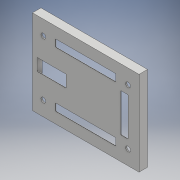
# Autodesk Inventor part: Platform-top
Saved by Autodesk Inventor 2017 (Build 210142000, 142)
## iProperties
Created: 2018-03-19
Part Number: Platform-top
Material: Generic
Document SubType Name: Modeling
Designer: Arjuna
Density: 1 g/cm^3
Appearance: Default
Author: Arjuna
Autodesk Inventor part; units mm, degrees
ref_plane "YZ Plane" through (0, 0, 0) normal (1, 0, 0) x (0, 1, 0)
ref_plane "XZ Plane" through (0, 0, 0) normal (0, 1, 0) x (-1, 0, 0)
ref_plane "XY Plane" through (0, 0, 0) normal (0, 0, 1) x (1, 0, 0)
sketch "Sketch1" plane through (0, 0, 0) normal (0, 1, 0) x (-1, 0, 0)
  line L0 (109.5, 87) -> (-109.5, 87)
  line L1 (-109.5, 87) -> (-109.5, -87)
  line L2 (-109.5, -87) -> (109.5, -87)
  line L3 (109.5, -87) -> (109.5, 87)
  point P0 (0, 0)
  dimension "d0" = 219
  dimension "d1" = 174
  dimension "d2" = 87
  dimension "d3" = 109.5
  constraints: 8 end point, 2 parallel, 1 horizontal, 1 perpendicular
  measures "d0" distance of L1.end L2.end
  measures "d1" distance of L2.end L0.start
  measures "d2" distance from line of point (0, 0) L0
  measures "d3" distance from line of point (0, 0) L1
extrude "Extrusion1" add sketch "Sketch1" along normal blind 17.5
sketch "Sketch2" plane through (0, 17.5, 0) normal (0, 1, 0) x (1, 0, 0)
  line L0 (-109.5, -87) -> (109.5, -87) projected
  line L1 (109.5, -87) -> (109.5, 87) projected
  line L2 (109.5, 87) -> (-109.5, 87) projected
  line L3 (-109.5, 87) -> (-109.5, -87) projected
  line L4 (-107, -84.5) -> (107, -84.5)
  line L5 (107, -84.5) -> (107, 84.5)
  line L6 (107, 84.5) -> (-107, 84.5)
  line L7 (-107, 84.5) -> (-107, -84.5)
  point P0 (0, 0)
  dimension "d6" = 2.5
  dimension "d7" = 2.5
  dimension "d8" = 2.5
  dimension "d9" = 2.5
  constraints: 8 end point, 2 parallel, 1 horizontal, 1 perpendicular
  measures "d6" distance between parallel lines of L3 L7
  measures "d7" distance between parallel lines of L2 L6
  measures "d8" distance between parallel lines of L0 L4
  measures "d9" distance between parallel lines of L1 L5
extrude "Extrusion2" cut sketch "Sketch2" against normal blind 15 contours L7 L6 L5 L4
sketch "Sketch3" plane through (0, 2.5, 0) normal (0, 1, 0) x (1, 0, 0)
  line L0 (-100, -12.5) -> (-40, -12.5)
  line L1 (-40, -12.5) -> (-40, 12.5)
  line L2 (-40, 12.5) -> (-100, 12.5)
  line L3 (-100, 12.5) -> (-100, -12.5)
  line L4 (-50, -19.5594) -> (-50, 30.4406)
  point P0 (0, 0)
  dimension "d12" = 60
  dimension "d13" = 25
  dimension "d14" = 12.5
  dimension "d15" = 40
  dimension "d16" = 50
  dimension "d17" = 50
  dimension "d18" = 50
  constraints: 10 end point, 2 parallel, 1 horizontal, 1 perpendicular, 1 vertical
  measures "d12" distance of L2.end L1.end
  measures "d13" distance of L2.end L0.start
  measures "d14" distance from line of point (0, 0) L0
  measures "d15" distance from line of point (0, 0) L1
  measures "d16" distance of L4.start L4.end
  measures "d17" distance from line of point (0, 0) L4
  measures "d18" distance between parallel lines of L4 L3
extrude "Extrusion3" cut sketch "Sketch3" against normal through all
sketch "Sketch4" plane through (0, 2.5, 0) normal (0, 1, 0) x (1, 0, 0)
  line L0 (-87, -64.5) -> (87, -64.5)
  line L1 (87, -64.5) -> (87, 64.5)
  line L2 (87, 64.5) -> (-87, 64.5)
  line L3 (-87, 64.5) -> (-87, -64.5)
  line L4 (-40, 12.5) -> (-40, -12.5) projected
  line L5 (-40, -12.5) -> (-100, -12.5) projected
  line L6 (-100, -12.5) -> (-100, 12.5) projected
  line L7 (-100, 12.5) -> (-40, 12.5) projected
  line L8 (107, -84.5) -> (-107, -84.5) projected
  line L9 (107, 84.5) -> (107, -84.5) projected
  line L10 (-107, 84.5) -> (107, 84.5) projected
  line L11 (-107, -84.5) -> (-107, 84.5) projected
  line L12 (-72, -49.5) -> (72, -49.5)
  line L13 (72, -49.5) -> (72, 49.5)
  line L14 (72, 49.5) -> (-72, 49.5)
  line L15 (-72, 49.5) -> (-72, -49.5)
  line L16 (-87, -39.5) -> (-72, -39.5)
  line L17 (-62, -49.5) -> (-62, -64.5)
  line L18 (-72, 39.5) -> (-87, 39.5)
  line L19 (-62, 49.5) -> (-62, 64.5)
  line L20 (62, 49.5) -> (62, 64.5)
  line L21 (72, 39.5) -> (87, 39.5)
  line L22 (72, -39.5) -> (87, -39.5)
  line L23 (62, -49.5) -> (62, -64.5)
  point P0 (0, 0)
  dimension "d21" = 20
  dimension "d22" = 20
  dimension "d23" = 20
  dimension "d24" = 20
  dimension "d25" = 15
  dimension "d26" = 15
  dimension "d27" = 15
  dimension "d28" = 15
  dimension "d29" = 25
  dimension "d30" = 25
  dimension "d31" = 25
  dimension "d32" = 25
  dimension "d33" = 25
  dimension "d34" = 25
  dimension "d35" = 25
  dimension "d36" = 25
  dimension "d169" = 129
  dimension "d170" = 174
  dimension "d171" = 87
  dimension "d172" = 64.5
  constraints: 32 end point, 16 point on line, 10 perpendicular, 4 parallel, 2 horizontal
  measures "d21" distance between parallel lines of L3 L11
  measures "d22" distance between parallel lines of L8 L0
  measures "d23" distance between parallel lines of L10 L2
  measures "d24" distance between parallel lines of L9 L1
  measures "d25" distance between parallel lines of L15 L3
  measures "d26" distance between parallel lines of L2 L14
  measures "d27" distance between parallel lines of L0 L12
  measures "d28" distance between parallel lines of L1 L13
  measures "d29" distance between parallel lines of L0 L16
  measures "d30" distance between parallel lines of L3 L17
  measures "d31" distance between parallel lines of L2 L18
  measures "d32" distance between parallel lines of L19 L3
  measures "d33" distance between parallel lines of L1 L20
  measures "d34" distance between parallel lines of L2 L21
  measures "d35" distance between parallel lines of L1 L23
  measures "d36" distance between parallel lines of L22 L0
  measures "d169" distance of L2.end L0.start
  measures "d170" distance of L0.start L0.end
  measures "d171" distance from line of point (0, 0) L3
  measures "d172" distance from line of point (0, 0) L0
extrude "Extrusion4" cut sketch "Sketch4" against normal through all contours L17 L12 L23 L0 | L22 L13 L21 L1 | L2 L20 L14 L19
sketch "Sketch5" plane through (0, 2.5, 0) normal (0, 1, 0) x (1, 0, 0)
  line L0 (62, -64.5) -> (-62, -64.5) projected
  line L1 (-62, -64.5) -> (-62, -49.5) projected
  line L2 (-62, -49.5) -> (62, -49.5) projected
  line L3 (62, -49.5) -> (62, -64.5) projected
  line L4 (87, -39.5) -> (72, -39.5) projected
  line L5 (72, -39.5) -> (72, 39.5) projected
  line L6 (72, 39.5) -> (87, 39.5) projected
  line L7 (87, 39.5) -> (87, -39.5) projected
  line L8 (62, 64.5) -> (62, 49.5) projected
  line L9 (62, 49.5) -> (-62, 49.5) projected
  line L10 (-62, 49.5) -> (-62, 64.5) projected
  line L11 (-62, 64.5) -> (62, 64.5) projected
  line L12 (-40, 12.5) -> (-40, -12.5) projected
  line L13 (-40, -12.5) -> (-100, -12.5) projected
  line L14 (-100, -12.5) -> (-100, 12.5) projected
  line L15 (-100, 12.5) -> (-40, 12.5) projected
  line L16 (107, -84.5) -> (-107, -84.5) projected
  line L17 (107, 84.5) -> (107, -84.5) projected
  line L18 (-107, 84.5) -> (107, 84.5) projected
  line L19 (-107, -84.5) -> (-107, 84.5) projected
  line L20 (-62, -62) -> (-72, -62)
  line L21 (-72, -62) -> (-72, -52)
  line L22 (-72, -52) -> (-62, -52)
  line L23 (-62, -52) -> (-62, -62)
  line L24 (62, -62) -> (72, -62)
  line L25 (72, -62) -> (72, -52)
  line L26 (72, -52) -> (62, -52)
  line L27 (62, -52) -> (62, -62)
  line L28 (84.5, -39.5) -> (74.5, -39.5)
  line L29 (74.5, -39.5) -> (74.5, -49.5)
  line L30 (74.5, -49.5) -> (84.5, -49.5)
  line L31 (84.5, -49.5) -> (84.5, -39.5)
  line L32 (74.5, 39.5) -> (84.5, 39.5)
  line L33 (84.5, 39.5) -> (84.5, 49.5)
  line L34 (84.5, 49.5) -> (74.5, 49.5)
  line L35 (74.5, 49.5) -> (74.5, 39.5)
  line L36 (-62, 52) -> (-72, 52)
  line L37 (-72, 52) -> (-72, 62)
  line L38 (-72, 62) -> (-62, 62)
  line L39 (-62, 62) -> (-62, 52)
  line L40 (62, 52) -> (72, 52)
  line L41 (72, 52) -> (72, 62)
  line L42 (72, 62) -> (62, 62)
  line L43 (62, 62) -> (62, 52)
  line L44 (-40, -10) -> (-30, -10)
  line L45 (-30, -10) -> (-30, 5)
  line L46 (-30, 5) -> (-40, 5)
  line L47 (-40, 5) -> (-40, -10)
  line L48 (-95, 12.5) -> (-45, 12.5)
  line L49 (-45, 12.5) -> (-45, 22.5)
  line L50 (-45, 22.5) -> (-95, 22.5)
  line L51 (-95, 22.5) -> (-95, 12.5)
  line L52 (-95, -12.5) -> (-45, -12.5)
  line L53 (-45, -12.5) -> (-45, -22.5)
  line L54 (-45, -22.5) -> (-95, -22.5)
  line L55 (-95, -22.5) -> (-95, -12.5)
  line L56 (-50, -49.5) -> (50, -49.5)
  line L57 (50, -49.5) -> (50, -39.5)
  line L58 (50, -39.5) -> (-50, -39.5)
  line L59 (-50, -39.5) -> (-50, -49.5)
  line L60 (-50, -64.5) -> (50, -64.5)
  line L61 (50, -64.5) -> (50, -74.5)
  line L62 (50, -74.5) -> (-50, -74.5)
  line L63 (-50, -74.5) -> (-50, -64.5)
  line L64 (-50, 49.5) -> (50, 49.5)
  line L65 (50, 49.5) -> (50, 39.5)
  line L66 (50, 39.5) -> (-50, 39.5)
  line L67 (-50, 39.5) -> (-50, 49.5)
  line L68 (-50, 64.5) -> (50, 64.5)
  line L69 (50, 64.5) -> (50, 74.5)
  line L70 (50, 74.5) -> (-50, 74.5)
  line L71 (-50, 74.5) -> (-50, 64.5)
  line L72 (72, -32.5) -> (62, -32.5)
  line L73 (62, -32.5) -> (62, 32.5)
  line L74 (62, 32.5) -> (72, 32.5)
  line L75 (72, 32.5) -> (72, -32.5)
  line L76 (87, -32.5) -> (97, -32.5)
  line L77 (97, -32.5) -> (97, 32.5)
  line L78 (97, 32.5) -> (87, 32.5)
  line L79 (87, 32.5) -> (87, -32.5)
  point P0 (0, 0)
  dimension "d39" = 10
  dimension "d40" = 10
  dimension "d41" = 2.5
  dimension "d42" = 2.5
  dimension "d43" = 10
  dimension "d44" = 10
  dimension "d45" = 2.5
  dimension "d46" = 2.5
  dimension "d47" = 10
  dimension "d48" = 10
  dimension "d49" = 2.5
  dimension "d50" = 2.5
  dimension "d51" = 10
  dimension "d52" = 10
  dimension "d53" = 2.5
  dimension "d54" = 2.5
  dimension "d55" = 10
  dimension "d56" = 10
  dimension "d57" = 2.5
  dimension "d58" = 10
  dimension "d59" = 10
  dimension "d60" = 2.5
  dimension "d61" = 2.5
  dimension "d62" = 10
  dimension "d63" = 15
  dimension "d64" = 2.5
  dimension "d65" = 7.5
  dimension "d66" = 50
  dimension "d67" = 10
  dimension "d68" = 5
  dimension "d69" = 5
  dimension "d70" = 50
  dimension "d71" = 10
  dimension "d72" = 5
  dimension "d73" = 5
  dimension "d74" = 100
  dimension "d75" = 10
  dimension "d76" = 12
  dimension "d77" = 12
  dimension "d78" = 100
  dimension "d79" = 10
  dimension "d80" = 12
  dimension "d81" = 12
  dimension "d82" = 100
  dimension "d83" = 10
  dimension "d84" = 12
  dimension "d85" = 12
  dimension "d86" = 100
  dimension "d87" = 10
  dimension "d88" = 12
  dimension "d89" = 12
  dimension "d90" = 65
  dimension "d91" = 10
  dimension "d92" = 7
  dimension "d93" = 7
  dimension "d94" = 10
  dimension "d95" = 65
  dimension "d96" = 7
  dimension "d97" = 7
  constraints: 120 end point, 30 parallel, 15 horizontal, 15 perpendicular, 15 point on line
  measures "d39" distance of L21.end L22.end
  measures "d40" distance of L20.end L21.end
  measures "d41" distance between parallel lines of L2 L22
  measures "d42" distance between parallel lines of L20 L0
  measures "d43" distance of L30.end L29.end
  measures "d44" distance of L28.end L29.end
  measures "d45" distance between parallel lines of L29 L5
  measures "d46" distance between parallel lines of L7 L31
  measures "d47" distance of L25.end L26.end
  measures "d48" distance of L24.end L25.end
  measures "d49" distance between parallel lines of L24 L0
  measures "d50" distance between parallel lines of L2 L26
  measures "d51" distance of L34.end L32.start
  measures "d52" distance of L33.end L34.end
  measures "d53" distance between parallel lines of L35 L5
  measures "d54" distance between parallel lines of L33 L7
  measures "d55" distance of L36.end L37.end
  measures "d56" distance of L37.end L38.end
  measures "d57" distance between parallel lines of L36 L9
  measures "d58" distance of L40.end L41.end
  measures "d59" distance of L41.end L42.end
  measures "d60" distance between parallel lines of L40 L9
  measures "d61" distance between parallel lines of L11 L42
  measures "d62" distance of L46.end L45.end
  measures "d63" distance of L44.end L45.end
  measures "d64" distance between parallel lines of L44 L13
  measures "d65" distance between parallel lines of L15 L46
  measures "d66" distance of L50.end L49.end
  measures "d67" distance of L50.end L48.start
  measures "d68" distance between parallel lines of L49 L12
  measures "d69" distance between parallel lines of L51 L14
  measures "d70" distance of L53.end L54.end
  measures "d71" distance of L54.end L52.start
  measures "d72" distance between parallel lines of L12 L53
  measures "d73" distance between parallel lines of L14 L55
  measures "d74" distance of L58.end L57.end
  measures "d75" distance of L58.end L56.start
  measures "d76" distance between parallel lines of L57 L3
  measures "d77" distance between parallel lines of L59 L1
  measures "d78" distance of L61.end L62.end
  measures "d79" distance of L62.end L60.start
  measures "d80" distance between parallel lines of L3 L61
  measures "d81" distance between parallel lines of L1 L63
  measures "d82" distance of L65.end L66.end
  measures "d83" distance of L66.end L64.start
  measures "d84" distance between parallel lines of L8 L65
  measures "d85" distance between parallel lines of L67 L10
  measures "d86" distance of L69.end L70.end
  measures "d87" distance of L70.end L68.start
  measures "d88" distance between parallel lines of L69 L8
  measures "d89" distance between parallel lines of L71 L10
  measures "d90" distance of L72.end L73.end
  measures "d91" distance of L73.end L74.end
  measures "d92" distance between parallel lines of L72 L4
  measures "d93" distance between parallel lines of L6 L74
  measures "d94" distance of L78.end L77.end
  measures "d95" distance of L76.end L77.end
  measures "d96" distance between parallel lines of L76 L4
  measures "d97" distance between parallel lines of L6 L78
extrude "Extrusion5" [suppressed]
sketch "Sketch6" plane through (0, 2.5, 0) normal (0, 1, 0) x (1, 0, 0)
  line L0 (-50, -74.5) -> (-50, -64.5) projected
  line L1 (50, -74.5) -> (-50, -74.5) projected
  line L2 (50, -64.5) -> (50, -74.5) projected
  line L3 (-50, -64.5) -> (50, -64.5) projected
  line L4 (-62, -52) -> (-62, -62) projected
  line L5 (-72, -52) -> (-62, -52) projected
  line L6 (-72, -62) -> (-72, -52) projected
  line L7 (-62, -62) -> (-72, -62) projected
  line L8 (50, -49.5) -> (-50, -49.5) projected
  line L9 (50, -39.5) -> (50, -49.5) projected
  line L10 (-50, -39.5) -> (50, -39.5) projected
  line L11 (-50, -49.5) -> (-50, -39.5) projected
  line L12 (72, -62) -> (62, -62) projected
  line L13 (72, -52) -> (72, -62) projected
  line L14 (62, -52) -> (72, -52) projected
  line L15 (62, -62) -> (62, -52) projected
  line L16 (-95, -20) -> (-95, -10) projected
  line L17 (-45, -20) -> (-95, -20) projected
  line L18 (-45, -10) -> (-45, -20) projected
  line L19 (-95, -10) -> (-45, -10) projected
  line L20 (-30, -7.5) -> (-40, -7.5) projected
  line L21 (-30, 7.5) -> (-30, -7.5) projected
  line L22 (-40, 7.5) -> (-30, 7.5) projected
  line L23 (-40, -7.5) -> (-40, 7.5) projected
  line L24 (-45, 10) -> (-95, 10) projected
  line L25 (-45, 20) -> (-45, 10) projected
  line L26 (-95, 20) -> (-45, 20) projected
  line L27 (-95, 10) -> (-95, 20) projected
  line L28 (-50, 39.5) -> (-50, 49.5) projected
  line L29 (50, 39.5) -> (-50, 39.5) projected
  line L30 (50, 49.5) -> (50, 39.5) projected
  line L31 (-50, 49.5) -> (50, 49.5) projected
  line L32 (-62, 62) -> (-62, 52) projected
  line L33 (-72, 62) -> (-62, 62) projected
  line L34 (-72, 52) -> (-72, 62) projected
  line L35 (-62, 52) -> (-72, 52) projected
  line L36 (50, 64.5) -> (-50, 64.5) projected
  line L37 (50, 74.5) -> (50, 64.5) projected
  line L38 (-50, 74.5) -> (50, 74.5) projected
  line L39 (-50, 64.5) -> (-50, 74.5) projected
  line L40 (72, 52) -> (62, 52) projected
  line L41 (72, 62) -> (72, 52) projected
  line L42 (62, 62) -> (72, 62) projected
  line L43 (62, 52) -> (62, 62) projected
  line L44 (72, 32.5) -> (72, -32.5) projected
  line L45 (72, 32.5) -> (72, -32.5) projected
  line L46 (62, 32.5) -> (72, 32.5) projected
  line L47 (62, -32.5) -> (62, 32.5) projected
  line L48 (72, -32.5) -> (62, -32.5) projected
  line L49 (74.5, -39.5) -> (84.5, -39.5) projected
  line L50 (74.5, -49.5) -> (74.5, -39.5) projected
  line L51 (84.5, -49.5) -> (74.5, -49.5) projected
  line L52 (84.5, -39.5) -> (84.5, -49.5) projected
  line L53 (97, -32.5) -> (87, -32.5) projected
  line L54 (97, 32.5) -> (97, -32.5) projected
  line L55 (87, 32.5) -> (97, 32.5) projected
  line L56 (87, -32.5) -> (87, 32.5) projected
  line L57 (84.5, 39.5) -> (74.5, 39.5) projected
  line L58 (84.5, 49.5) -> (84.5, 39.5) projected
  line L59 (74.5, 49.5) -> (84.5, 49.5) projected
  line L60 (74.5, 39.5) -> (74.5, 49.5) projected
  line L61 (-62, -62) -> (-64.5, -62)
  line L62 (-64.5, -62) -> (-64.5, -52)
  line L63 (-64.5, -52) -> (-62, -52)
  line L64 (-62, -52) -> (-62, -62)
  line L65 (-50, -49.5) -> (50, -49.5)
  line L66 (50, -49.5) -> (50, -47)
  line L67 (50, -47) -> (-50, -47)
  line L68 (-50, -47) -> (-50, -49.5)
  line L69 (50, -64.5) -> (-50, -64.5)
  line L70 (-50, -64.5) -> (-50, -67)
  line L71 (-50, -67) -> (50, -67)
  line L72 (50, -67) -> (50, -64.5)
  line L73 (62, -62) -> (64.5, -62)
  line L74 (64.5, -62) -> (64.5, -52)
  line L75 (64.5, -52) -> (62, -52)
  line L76 (62, -52) -> (62, -62)
  line L77 (72, -32.5) -> (69.5, -32.5)
  line L78 (69.5, -32.5) -> (69.5, 32.5)
  line L79 (69.5, 32.5) -> (72, 32.5)
  line L80 (72, 32.5) -> (72, -32.5)
  line L81 (74.5, -39.5) -> (84.5, -39.5)
  line L82 (84.5, -39.5) -> (84.5, -42)
  line L83 (84.5, -42) -> (74.5, -42)
  line L84 (74.5, -42) -> (74.5, -39.5)
  line L85 (87, -32.5) -> (89.5, -32.5)
  line L86 (89.5, -32.5) -> (89.5, 32.5)
  line L87 (89.5, 32.5) -> (87, 32.5)
  line L88 (87, 32.5) -> (87, -32.5)
  line L89 (84.5, 39.5) -> (74.5, 39.5)
  line L90 (74.5, 39.5) -> (74.5, 42)
  line L91 (74.5, 42) -> (84.5, 42)
  line L92 (84.5, 42) -> (84.5, 39.5)
  line L93 (-62, 52) -> (-64.5, 52)
  line L94 (-64.5, 52) -> (-64.5, 62)
  line L95 (-64.5, 62) -> (-62, 62)
  line L96 (-62, 62) -> (-62, 52)
  line L97 (-50, 64.5) -> (50, 64.5)
  line L98 (50, 64.5) -> (50, 67)
  line L99 (50, 67) -> (-50, 67)
  line L100 (-50, 67) -> (-50, 64.5)
  line L101 (-50, 49.5) -> (50, 49.5)
  line L102 (50, 49.5) -> (50, 47)
  line L103 (50, 47) -> (-50, 47)
  line L104 (-50, 47) -> (-50, 49.5)
  line L105 (62, 52) -> (64.5, 52)
  line L106 (64.5, 52) -> (64.5, 62)
  line L107 (64.5, 62) -> (62, 62)
  line L108 (62, 62) -> (62, 52)
  line L109 (-40, -7.5) -> (-37.5, -7.5)
  line L110 (-37.5, -7.5) -> (-37.5, 7.5)
  line L111 (-37.5, 7.5) -> (-40, 7.5)
  line L112 (-40, 7.5) -> (-40, -7.5)
  line L113 (-45, -10) -> (-95, -10)
  line L114 (-95, -10) -> (-95, -12.5)
  line L115 (-95, -12.5) -> (-45, -12.5)
  line L116 (-45, -12.5) -> (-45, -10)
  line L117 (-45, 10) -> (-95, 10)
  line L118 (-95, 10) -> (-95, 12.5)
  line L119 (-95, 12.5) -> (-45, 12.5)
  line L120 (-45, 12.5) -> (-45, 10)
  circle A0 centre (-68, -57) radius 1.5
  circle A1 centre (-42.5, -70.5) radius 1.5
  circle A2 centre (42.5, -70.5) radius 1.5
  circle A3 centre (-42.5, -43.5) radius 1.5
  circle A4 centre (42.5, -43.5) radius 1.5
  circle A5 centre (68, -57) radius 1.5
  circle A6 centre (-90, -16) radius 1.5
  circle A7 centre (-50, -16) radius 1.5
  circle A8 centre (79.5, -45.5) radius 1.5
  circle A9 centre (-34, 0) radius 1.5
  circle A10 centre (66, -27.5) radius 1.5
  circle A11 centre (93, -27.5) radius 1.5
  line L121 (-124.5472, 0) -> (126.6458, 0)
  circle A12 centre (-68, 57) radius 1.5
  circle A13 centre (-42.5, 70.5) radius 1.5
  circle A14 centre (42.5, 70.5) radius 1.5
  circle A15 centre (-42.5, 43.5) radius 1.5
  circle A16 centre (42.5, 43.5) radius 1.5
  circle A17 centre (68, 57) radius 1.5
  circle A18 centre (-90, 16) radius 1.5
  circle A19 centre (-50, 16) radius 1.5
  circle A20 centre (79.5, 45.5) radius 1.5
  circle A21 centre (66, 27.5) radius 1.5
  circle A22 centre (93, 27.5) radius 1.5
  point P0 (0, 0)
  dimension "d100" = 2.5
  dimension "d101" = 2.5
  dimension "d102" = 2.5
  dimension "d103" = 2.5
  dimension "d104" = 2.5
  dimension "d105" = 2.5
  dimension "d106" = 2.5
  dimension "d107" = 2.5
  dimension "d108" = 2.5
  dimension "d109" = 2.5
  dimension "d110" = 2.5
  dimension "d111" = 2.5
  dimension "d112" = 2.5
  dimension "d113" = 2.5
  dimension "d114" = 2.5
  dimension "d117" = 3
  dimension "d118" = 4
  dimension "d119" = 5
  dimension "d120" = 3
  dimension "d121" = 4
  dimension "d122" = 7.5
  dimension "d123" = 3
  dimension "d124" = 7.5
  dimension "d125" = 4
  dimension "d126" = 3
  dimension "d127" = 7.5
  dimension "d128" = 4
  dimension "d129" = 3
  dimension "d130" = 4
  dimension "d131" = 7.5
  dimension "d132" = 3
  dimension "d133" = 5
  dimension "d134" = 4
  dimension "d135" = 3
  dimension "d136" = 4
  dimension "d137" = 5
  dimension "d138" = 3
  dimension "d139" = 4
  dimension "d140" = 5
  dimension "d141" = 3
  dimension "d142" = 5
  dimension "d143" = 4
  dimension "d144" = 3
  dimension "d145" = 4
  dimension "d146" = 7.5
  dimension "d147" = 3
  dimension "d148" = 4
  dimension "d149" = 5
  dimension "d150" = 3
  dimension "d151" = 4
  dimension "d152" = 5
  constraints: 122 end point, 30 parallel, 23 centre point, 16 horizontal, 15 perpendicular, 15 point on line, 11 symmetric about line, 11 other
  measures "d100" distance of L62.end L63.end
  measures "d101" distance between parallel lines of L67 L8
  measures "d102" distance between parallel lines of L3 L71
  measures "d103" distance of L75.end L74.end
  measures "d104" distance of L78.end L79.end
  measures "d105" distance of L87.end L86.end
  measures "d106" distance of L83.end L49.start
  measures "d107" distance of L89.end L90.end
  measures "d108" distance between parallel lines of L19 L115
  measures "d109" distance between parallel lines of L110 L112
  measures "d110" distance between parallel lines of L119 L24
  measures "d111" distance between parallel lines of L32 L94
  measures "d112" distance between parallel lines of L101 L103
  measures "d113" distance between parallel lines of L99 L36
  measures "d114" distance between parallel lines of L106 L43
  measures "d117" diameter of A0
  measures "d118" distance from line of A0.centre L6
  measures "d119" distance from line of L5 A0.centre
  measures "d120" diameter of A1
  measures "d121" distance from line of A1.centre L1
  measures "d122" distance from line of L0 A1.centre
  measures "d123" diameter of A2
  measures "d124" distance from line of L2 A2.centre
  measures "d125" distance from line of L1 A2.centre
  measures "d126" diameter of A3
  measures "d127" distance from line of A3.centre L11
  measures "d128" distance from line of L10 A3.centre
  measures "d129" diameter of A4
  measures "d130" distance from line of L10 A4.centre
  measures "d131" distance from line of L9 A4.centre
  measures "d132" diameter of A5
  measures "d133" distance from line of L14 A5.centre
  measures "d134" distance from line of L13 A5.centre
  measures "d135" diameter of A6
  measures "d136" distance from line of L17 A6.centre
  measures "d137" distance from line of A6.centre L16
  measures "d138" diameter of A7
  measures "d139" distance from line of L17 A7.centre
  measures "d140" distance from line of L18 A7.centre
  measures "d141" diameter of A8
  measures "d142" distance from line of A8.centre L50
  measures "d143" distance from line of L51 A8.centre
  measures "d144" diameter of A9
  measures "d145" distance from line of L21 A9.centre
  measures "d146" distance from line of L20 A9.centre
  measures "d147" diameter of A10
  measures "d148" distance from line of A10.centre L47
  measures "d149" distance from line of L48 A10.centre
  measures "d150" diameter of A11
  measures "d151" distance from line of L54 A11.centre
  measures "d152" distance from line of L53 A11.centre
extrude "Extrusion6" [suppressed]
sketch "Sketch7" plane through (0, 2.5, 0) normal (0, 1, 0) x (1, 0, 0)
  line L0 (62, -64.5) -> (-62, -64.5) projected
  line L1 (-62, -64.5) -> (-62, -49.5) projected
  line L2 (-62, -49.5) -> (62, -49.5) projected
  line L3 (62, -49.5) -> (62, -64.5) projected
  line L4 (87, -39.5) -> (72, -39.5) projected
  line L5 (72, -39.5) -> (72, 39.5) projected
  line L6 (72, 39.5) -> (87, 39.5) projected
  line L7 (87, 39.5) -> (87, -39.5) projected
  line L8 (62, 64.5) -> (62, 49.5) projected
  line L9 (62, 49.5) -> (-62, 49.5) projected
  line L10 (-62, 49.5) -> (-62, 64.5) projected
  line L11 (-62, 64.5) -> (62, 64.5) projected
  line L12 (-40, 12.5) -> (-40, -12.5) projected
  line L13 (-40, -12.5) -> (-100, -12.5) projected
  line L14 (-100, -12.5) -> (-100, 12.5) projected
  line L15 (-100, 12.5) -> (-40, 12.5) projected
  line L16 (107, -84.5) -> (-107, -84.5) projected
  line L17 (107, 84.5) -> (107, -84.5) projected
  line L18 (-107, 84.5) -> (107, 84.5) projected
  line L19 (-107, -84.5) -> (-107, 84.5) projected
  circle A0 centre (-87, -57) radius 5
  circle A1 centre (-87, 57) radius 5
  circle A2 centre (87, -57) radius 5
  circle A3 centre (87, 57) radius 5
  point P0 (0, 0)
  dimension "d153" = 10
  dimension "d154" = 20
  dimension "d155" = 27.5
  dimension "d156" = 10
  dimension "d157" = 20
  dimension "d158" = 27.5
  dimension "d159" = 10
  dimension "d160" = 20
  dimension "d161" = 27.5
  dimension "d162" = 10
  dimension "d163" = 20
  dimension "d164" = 27.5
  dimension "d167" = 87
  dimension "d168" = 57
  constraints: 4 centre point
  measures "d153" diameter of A0
  measures "d154" distance from line of L19 A0.centre
  measures "d155" distance from line of L16 A0.centre
  measures "d156" diameter of A1
  measures "d157" distance from line of L19 A1.centre
  measures "d158" distance from line of L18 A1.centre
  measures "d159" diameter of A2
  measures "d160" distance from line of L17 A2.centre
  measures "d161" distance from line of L16 A2.centre
  measures "d162" diameter of A3
  measures "d163" distance from line of L17 A3.centre
  measures "d164" distance from line of L18 A3.centre
  measures "d167" horizontal distance of point (0, 0) A0.centre
  measures "d168" vertical distance of point (0, 0) A0.centre
extrude "Extrusion7" cut sketch "Sketch7" against normal through all contours A0 | A1 | A2 | A3
fillet "Fillet1" radius 2 16 edges at (-70, 2.5, 12.5) (-100, 2.5, 0) (-70, 2.5, -12.5) (-40, 2.5, 0) (-62, 2.5, 57) (0, 2.5, 64.5) (0, 2.5, 49.5) (62, 2.5, 57) (72, 2.5, 0) (79.5, 2.5, 39.5) (87, 2.5, 0) (79.5, 2.5, -39.5) (0, 2.5, -49.5) (62, 2.5, -57) (0, 2.5, -64.5) (-62, 2.5, -57)
fillet "Fillet2" radius 1 32 edges at (-40, 0.25, 12.5) (-39.4142, 1.9142, 13.0858) (-100, 0.25, 12.5) (-100.5858, 1.9142, 13.0858) (-100, 0.25, -12.5) (-100.5858, 1.9142, -13.0858) (-40, 0.25, -12.5) (-39.4142, 1.9142, -13.0858) (-62, 0.25, -49.5) (-62.5858, 1.9142, -48.9142) (-62, 0.25, -64.5) (-62.5858, 1.9142, -65.0858) (62, 0.25, -49.5) (62.5858, 1.9142, -48.9142) (62, 0.25, -64.5) (62.5858, 1.9142, -65.0858) (72, 0.25, -39.5) (71.4142, 1.9142, -40.0858) (72, 0.25, 39.5) (71.4142, 1.9142, 40.0858) (87, 0.25, 39.5) (87.5858, 1.9142, 40.0858) (87, 0.25, -39.5) (87.5858, 1.9142, -40.0858) (62, 0.25, 64.5) (62.5858, 1.9142, 65.0858) (62, 0.25, 49.5) (62.5858, 1.9142, 48.9142) (-62, 0.25, 64.5) (-62.5858, 1.9142, 65.0858) (-62, 0.25, 49.5) (-62.5858, 1.9142, 48.9142)
equation "\"d2\" = 0.5 * d1"
equation "\"d3\" = 0.5 * d0"
equation "\"d7\" = d6"
equation "\"d8\" = d6"
equation "\"d9\" = d6"
equation "\"d14\" = 0.5 * d13"
equation "\"d22\" = d21"
equation "\"d23\" = d21"
equation "\"d24\" = d21"
equation "\"d26\" = d25"
equation "\"d27\" = d25"
equation "\"d28\" = d25"
equation "\"d30\" = d29"
equation "\"d31\" = d29"
equation "\"d32\" = d29"
equation "\"d33\" = d29"
equation "\"d34\" = d29"
equation "\"d35\" = d29"
equation "\"d36\" = d29"
equation "\"d43\" = d40"
equation "\"d44\" = d39"
equation "\"d45\" = d41"
equation "\"d47\" = d39"
equation "\"d48\" = d40"
equation "\"d49\" = d41"
equation "\"d51\" = d39"
equation "\"d52\" = d40"
equation "\"d53\" = d41"
equation "\"d55\" = d40"
equation "\"d56\" = d39"
equation "\"d57\" = d41"
equation "\"d58\" = d40"
equation "\"d59\" = d39"
equation "\"d60\" = d41"
equation "\"d70\" = d66"
equation "\"d71\" = d67"
equation "\"d72\" = d68"
equation "\"d78\" = d74"
equation "\"d79\" = d75"
equation "\"d80\" = d76"
equation "\"d82\" = d74"
equation "\"d83\" = d75"
equation "\"d84\" = d76"
equation "\"d86\" = d74"
equation "\"d87\" = d75"
equation "\"d88\" = d76"
equation "\"d94\" = d91"
equation "\"d95\" = d90"
equation "\"d96\" = d92"
equation "\"d101\" = d100"
equation "\"d102\" = d100"
equation "\"d103\" = d100"
equation "\"d104\" = d100"
equation "\"d105\" = d100"
equation "\"d106\" = d100"
equation "\"d107\" = d100"
equation "\"d108\" = d100"
equation "\"d109\" = d100"
equation "\"d110\" = d100"
equation "\"d111\" = d100"
equation "\"d112\" = d100"
equation "\"d113\" = d100"
equation "\"d114\" = d100"
equation "\"d120\" = d117"
equation "\"d121\" = d118"
equation "\"d123\" = d117"
equation "\"d124\" = d122"
equation "\"d125\" = d118"
equation "\"d126\" = d117"
equation "\"d127\" = d122"
equation "\"d128\" = d118"
equation "\"d129\" = d117"
equation "\"d130\" = d118"
equation "\"d131\" = d122"
equation "\"d132\" = d117"
equation "\"d133\" = d119"
equation "\"d134\" = d118"
equation "\"d135\" = d117"
equation "\"d136\" = d118"
equation "\"d138\" = d117"
equation "\"d139\" = d118"
equation "\"d140\" = d137"
equation "\"d141\" = d117"
equation "\"d142\" = d119"
equation "\"d143\" = d118"
equation "\"d144\" = d117"
equation "\"d145\" = d118"
equation "\"d147\" = d117"
equation "\"d148\" = d118"
equation "\"d150\" = d117"
equation "\"d151\" = d118"
equation "\"d152\" = d149"
equation "\"d156\" = d153"
equation "\"d157\" = d154"
equation "\"d158\" = d155"
equation "\"d159\" = d153"
equation "\"d160\" = d154"
equation "\"d161\" = d155"
equation "\"d162\" = d153"
equation "\"d163\" = d154"
equation "\"d164\" = d155"
body "Solid1"
